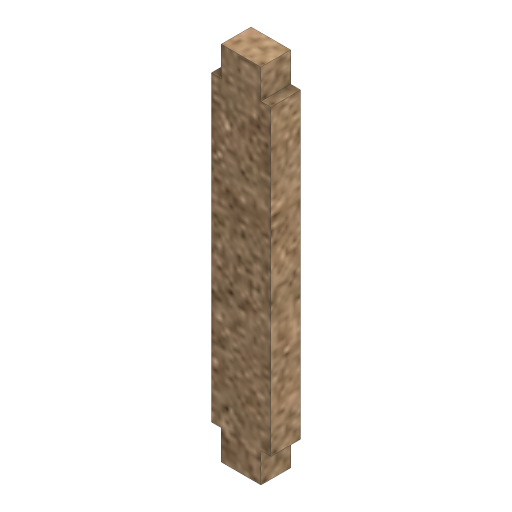
# Autodesk Inventor part: final_side_hold_3
Saved by Autodesk Inventor 2024 (Build 280153000, 153)
## iProperties
Created: 2024-05-27
Material: MDF Medium Density Fiberboard
Document SubType Name: Modeling
Designer: op04o
Density: 0.8 g/cm^3
Appearance: Cardboard - Corrugated
Mass: 0.496944 g
Surface Area: 6.6918 cm^2
Volume: 0.62118 cm^3
Author: 第26組
Title: final_side_hold_3
Autodesk Inventor part; units mm, degrees
ref_plane "YZ Plane" through (0, 0, 0) normal (1, 0, 0) x (0, 1, 0)
ref_plane "XZ Plane" through (0, 0, 0) normal (0, 1, 0) x (-1, 0, 0)
ref_plane "XY Plane" through (0, 0, 0) normal (0, 0, 1) x (1, 0, 0)
sketch "Sketch1" plane through (0, 0, 0) normal (0, 0, 1) x (1, 0, 0)
  line L0 (-3, 15.255) -> (3, 15.255)
  line L1 (3, 15.255) -> (3, -15.255)
  line L2 (3, -15.255) -> (-3, -15.255)
  line L3 (-3, -15.255) -> (-3, 15.255)
  line L4 (-2, -15.255) -> (2, -15.255)
  line L5 (2, -15.255) -> (2, -18.255)
  line L6 (2, -18.255) -> (-2, -18.255)
  line L7 (-2, -18.255) -> (-2, -15.255)
  line L8 (-2, 15.255) -> (2, 15.255)
  line L9 (2, 15.255) -> (2, 18.255)
  line L10 (2, 18.255) -> (-2, 18.255)
  line L11 (-2, 18.255) -> (-2, 15.255)
  line L12 (3, -12) -> (0, -12)
  line L13 (0, -12) -> (0, -8)
  line L14 (0, -8) -> (3, -8)
  line L15 (3, -8) -> (3, -12)
  line L16 (3, 8) -> (0, 8)
  line L17 (0, 8) -> (0, 12)
  line L18 (0, 12) -> (3, 12)
  line L19 (3, 12) -> (3, 8)
  point P0 (0, 0)
  point P1 (0, 0)
  point P2 (0, 18.255)
  point P3 (0, 15.255)
  point P4 (0, 15.255)
  point P5 (0, -18.255)
  point P6 (3, 0)
  point P7 (2.1852, -20.4852)
  point P8 (2.1852, 20.1148)
  point P9 (3, -10)
  point P10 (3, 10)
  point P11 (3.1852, -8.1852)
  point P12 (3.1852, 11.8148)
  dimension "d0" = 36.51
  dimension "d1" = 3
  dimension "d2" = 4
  dimension "d3" = 6
  dimension "d4" = 4
  dimension "d5" = 10
  dimension "d6" = 10
  dimension "d7" = 3
  constraints: 40 end point, 10 parallel, 7 midpoint, 6 point on line, 5 horizontal, 5 perpendicular, 3 vertical alignment, 2 collinear, 1 coincident, 1 horizontal alignment
  measures "d0" distance between parallel lines of L6 L10
  measures "d1" distance of L8.end L9.end
  measures "d2" distance of L9.end L10.end
  measures "d3" distance of L0.start L0.end
  measures "d4" distance of L12.end L13.end
  measures "d5" distance of point (3, 0) point (3, -10)
  measures "d6" distance of point (3, 10) point (3, 0)
  measures "d7" distance of L13.end L14.end
extrude "Extrusion1" add sketch "Sketch1" along normal blind 3
body "Solid1"
